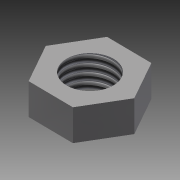
# Autodesk Inventor part: 3asAnya
Saved by Autodesk Inventor 2015 (Build 190159000, 159)
## iProperties
Created: 2014-11-03
Part Number: 3asAnya
Material: Steel, Alloy
Document SubType Name: Modeling
Designer: laca
Density: 7.73 g/cm^3
Appearance: Semi-Polished
Mass: 0.225439 g
Surface Area: 0.826547 cm^2
Volume: 0.0291641 cm^3
Author: laca
Autodesk Inventor part; units mm, degrees
ref_plane "YZ Plane" through (0, 0, 0) normal (1, 0, 0) x (0, 1, 0)
ref_plane "XZ Plane" through (0, 0, 0) normal (0, 1, 0) x (-1, 0, 0)
ref_plane "XY Plane" through (0, 0, 0) normal (0, 0, 1) x (1, 0, 0)
sketch "Sketch1" plane through (0, 0, 0) normal (0, 1, 0) x (-1, 0, 0)
  line L0 (1.4722, 2.4832) -> (2.8866, -0.0333)
  line L1 (2.8866, -0.0333) -> (1.4144, -2.5165)
  line L2 (1.4144, -2.5165) -> (-1.4722, -2.4832)
  line L3 (-1.4722, -2.4832) -> (-2.8866, 0.0333)
  line L4 (-2.8866, 0.0333) -> (-1.4144, 2.5165)
  line L5 (-1.4144, 2.5165) -> (1.4722, 2.4832)
  circle A0 centre (0, 0) radius 1.5
  dimension "d0" = 5
  dimension "d1" = 3
  constraints: 12 end point, 2 coincident, 1 centre point, 13 other
  measures "d0" distance between parallel lines of L2 L5
  measures "d1" diameter of A0
extrude "Extrusion1" add sketch "Sketch1" along normal blind 2
thread "Thread1" size "M3x0.5" class "6H" standard "ANSI Metric M Profile" full length
body "Solid1"
